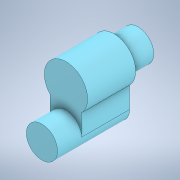
# Autodesk Inventor part: Component29
Saved by Autodesk Inventor 2022 (Build 260153000, 153)
## iProperties
Created: 2022-01-29
Part Number: Component29
Material: Generic
Document SubType Name: Modeling
Designer: Administrator
Density: 1 g/cm^3
Appearance: Default
Title: Component29
Author: Administrator
Autodesk Inventor part; units mm, degrees
ref_plane "YZ Plane" through (0, 0, 0) normal (1, 0, 0) x (0, 1, 0)
ref_plane "XZ Plane" through (0, 0, 0) normal (0, 1, 0) x (-1, 0, 0)
ref_plane "XY Plane" through (0, 0, 0) normal (0, 0, 1) x (1, 0, 0)
sketch "Sketch2" plane through (0, 0, 0) normal (0, 0, 1) x (1, 0, 0)
  line L0 (1.043, 0.3192) -> (1.043, -4.0683)
  arc A0 (1.043, 0.3192) -> (-5.457, 0.3192) centre (-2.207, 3.4317) ccw
  circle A1 centre (-2.207, -4.0683) radius 3.25
  circle A2 centre (-2.207, 3.4317) radius 3.25
  line L1 (-2.207, 14.5026) -> (-2.207, -15.0875) construction
  line L2 (-5.457, 0.3192) -> (-5.457, -4.0683)
  point P0 (-2.7063, -6.309)
  dimension "d6" = 6.5
  dimension "d8" = 9
  dimension "d9" = 7.5
  constraints: 6 end point, 3 vertical, 2 centre point, 2 point on circle, 2 point on line, 2 symmetric about line, 1 coincident, 1 parallel, 4 other
  measures "d8" diameter of A0
  measures "d9" distance of point (-2.207, -4.068) A0.centre
extrude "Extrusion1" add sketch "Sketch2" along normal blind 5 contours A1
extrude "Extrusion2" add sketch "Sketch2" against normal blind 10 contours L0 A1 L2 A0 | A1 | A2
sketch "Sketch3" plane through (0, 0, -10) normal (0, 0, -1) x (-1, 0, 0)
  circle A0 centre (2.207, 3.4317) radius 3.25 projected
  arc A1 (5.457, 0.3192) -> (-1.043, 0.3192) centre (2.207, 3.4317) ccw projected
  point P0 (0, 0)
extrude "Extrusion3" add sketch "Sketch3" along normal blind 5
equation "\"d6\" = R"
equation "\"d8\" = R1"
equation "\"d0\" = thickness"
equation "\"d2\" = 2 * thickness"
equation "\"d4\" = thickness"
equation "\"R\" = 6.5"
equation "\"thickness\" = 5"
equation "\"width\" = 6.5"
equation "\"R1\" = 9"
body "Solid1"
